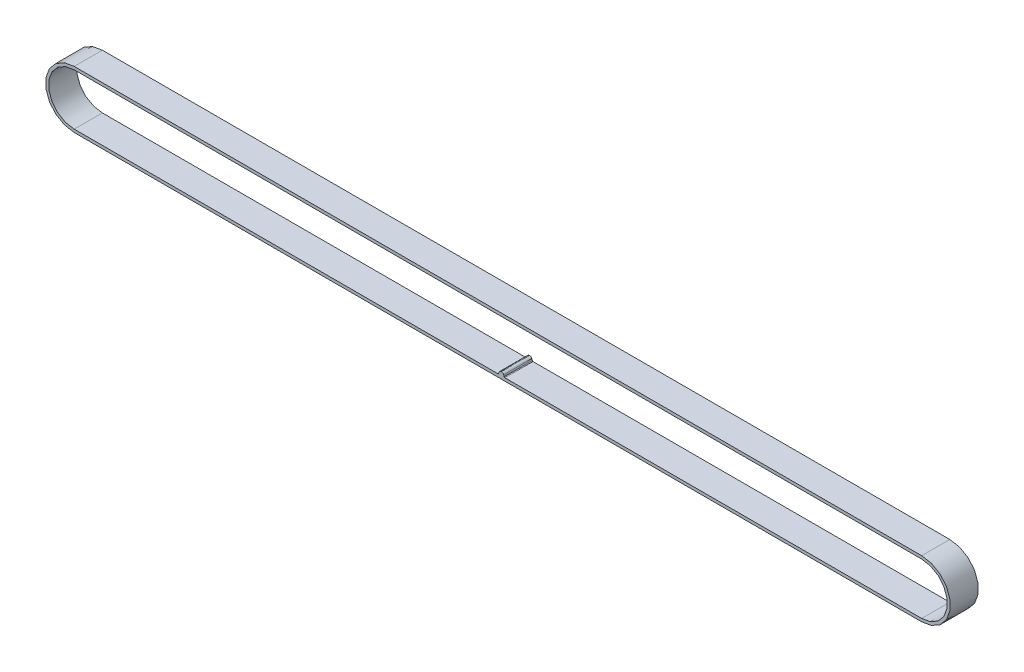
# Autodesk Inventor part: correia
Saved by Autodesk Inventor 2023 (Build 270158000, 158)
## iProperties
Created: 2022-10-19
Part Number: correia
Material: Generic
Document SubType Name: Modeling
Designer: klebe
Density: 1 g/cm^3
Appearance: Default
Author: klebe
Autodesk Inventor part; units mm, degrees
(part 1 of 6)
ref_plane "YZ Plane" through (0, 0, 0) normal (1, 0, 0) x (0, 1, 0)
ref_plane "XZ Plane" through (0, 0, 0) normal (0, 1, 0) x (-1, 0, 0)
ref_plane "XY Plane" through (0, 0, 0) normal (0, 0, 1) x (1, 0, 0)
ref_plane "Work Plane2" through (-56.6424, 85.638, -97) normal (0, 0, 1) x (-1, 0, 0)
sketch "Sketch2" plane through (-56.6424, 85.638, -97) normal (0, 0, 1) x (-1, 0, 0)
  arc A0 (0, 0) -> (0, 50.63) centre (0, 25.315) ccw
  line L0 (-421.46, 50.63) -> (0, 50.63)
  arc A1 (-421.46, 50.63) -> (-421.46, 0) centre (-421.46, 25.315) ccw
  line L1 (0, 0) -> (-421.46, 0)
  arc A2 (-204.9902, 50) -> (-205.1389, 49.8696) centre (-204.9902, 49.85) ccw
  line L2 (-204.9902, 50) -> (-204.4709, 50)
  arc A3 (-204.3222, 49.8696) -> (-204.4709, 50) centre (-204.4709, 49.85) ccw
  arc A4 (-204.3222, 49.8696) -> (-204.2296, 49.5618) centre (-203.3307, 50) ccw
  arc A5 (-204.2296, 49.5618) -> (-203.7306, 49.25) centre (-203.7307, 49.805) ccw
  arc A6 (-203.7306, 49.25) -> (-203.2315, 49.5618) centre (-203.7304, 49.805) ccw
  arc A7 (-203.2315, 49.5618) -> (-203.1389, 49.8696) centre (-204.1304, 50) ccw
  arc A8 (-202.9902, 50) -> (-203.1389, 49.8696) centre (-202.9902, 49.85) ccw
  line L3 (-202.9902, 50) -> (-202.4709, 50)
  arc A9 (-202.3222, 49.8696) -> (-202.4709, 50) centre (-202.4709, 49.85) ccw
  arc A10 (-202.3222, 49.8696) -> (-202.2296, 49.5618) centre (-201.3307, 50) ccw
  arc A11 (-202.2296, 49.5618) -> (-201.7306, 49.25) centre (-201.7307, 49.805) ccw
  arc A12 (-201.7306, 49.25) -> (-201.2315, 49.5618) centre (-201.7304, 49.805) ccw
  arc A13 (-201.2315, 49.5618) -> (-201.1389, 49.8696) centre (-202.1304, 50) ccw
  arc A14 (-200.9902, 50) -> (-201.1389, 49.8696) centre (-200.9902, 49.85) ccw
  line L4 (-200.9902, 50) -> (-200.4709, 50)
  arc A15 (-200.3222, 49.8696) -> (-200.4709, 50) centre (-200.4709, 49.85) ccw
  arc A16 (-200.3222, 49.8696) -> (-200.2296, 49.5618) centre (-199.3307, 50) ccw
  arc A17 (-200.2296, 49.5618) -> (-199.7306, 49.25) centre (-199.7307, 49.805) ccw
  arc A18 (-199.7306, 49.25) -> (-199.2315, 49.5618) centre (-199.7304, 49.805) ccw
  arc A19 (-199.2315, 49.5618) -> (-199.1389, 49.8696) centre (-200.1304, 50) ccw
  arc A20 (-198.9902, 50) -> (-199.1389, 49.8696) centre (-198.9902, 49.85) ccw
  line L5 (-198.9902, 50) -> (-198.4709, 50)
  arc A21 (-198.3222, 49.8696) -> (-198.4709, 50) centre (-198.4709, 49.85) ccw
  arc A22 (-198.3222, 49.8696) -> (-198.2296, 49.5618) centre (-197.3307, 50) ccw
  arc A23 (-198.2296, 49.5618) -> (-197.7306, 49.25) centre (-197.7307, 49.805) ccw
  arc A24 (-197.7306, 49.25) -> (-197.2315, 49.5618) centre (-197.7304, 49.805) ccw
  arc A25 (-197.2315, 49.5618) -> (-197.1389, 49.8696) centre (-198.1304, 50) ccw
  arc A26 (-196.9902, 50) -> (-197.1389, 49.8696) centre (-196.9902, 49.85) ccw
  line L6 (-196.9902, 50) -> (-196.4709, 50)
  arc A27 (-196.3222, 49.8696) -> (-196.4709, 50) centre (-196.4709, 49.85) ccw
  arc A28 (-196.3222, 49.8696) -> (-196.2296, 49.5618) centre (-195.3307, 50) ccw
  arc A29 (-196.2296, 49.5618) -> (-195.7306, 49.25) centre (-195.7307, 49.805) ccw
  arc A30 (-195.7306, 49.25) -> (-195.2315, 49.5618) centre (-195.7304, 49.805) ccw
  arc A31 (-195.2315, 49.5618) -> (-195.1389, 49.8696) centre (-196.1304, 50) ccw
  arc A32 (-194.9902, 50) -> (-195.1389, 49.8696) centre (-194.9902, 49.85) ccw
  line L7 (-194.9902, 50) -> (-194.4709, 50)
  arc A33 (-194.3222, 49.8696) -> (-194.4709, 50) centre (-194.4709, 49.85) ccw
  arc A34 (-194.3222, 49.8696) -> (-194.2296, 49.5618) centre (-193.3307, 50) ccw
  arc A35 (-194.2296, 49.5618) -> (-193.7306, 49.25) centre (-193.7307, 49.805) ccw
  arc A36 (-193.7306, 49.25) -> (-193.2315, 49.5618) centre (-193.7304, 49.805) ccw
  arc A37 (-193.2315, 49.5618) -> (-193.1389, 49.8696) centre (-194.1304, 50) ccw
  arc A38 (-192.9902, 50) -> (-193.1389, 49.8696) centre (-192.9902, 49.85) ccw
  line L8 (-192.9902, 50) -> (-192.4709, 50)
  arc A39 (-192.3222, 49.8696) -> (-192.4709, 50) centre (-192.4709, 49.85) ccw
  arc A40 (-192.3222, 49.8696) -> (-192.2296, 49.5618) centre (-191.3307, 50) ccw
  arc A41 (-192.2296, 49.5618) -> (-191.7306, 49.25) centre (-191.7307, 49.805) ccw
  arc A42 (-191.7306, 49.25) -> (-191.2315, 49.5618) centre (-191.7304, 49.805) ccw
  arc A43 (-191.2315, 49.5618) -> (-191.1389, 49.8696) centre (-192.1304, 50) ccw
  arc A44 (-190.9902, 50) -> (-191.1389, 49.8696) centre (-190.9902, 49.85) ccw
  line L9 (-190.9902, 50) -> (-190.4709, 50)
  arc A45 (-190.3222, 49.8696) -> (-190.4709, 50) centre (-190.4709, 49.85) ccw
  arc A46 (-190.3222, 49.8696) -> (-190.2296, 49.5618) centre (-189.3307, 50) ccw
  arc A47 (-190.2296, 49.5618) -> (-189.7306, 49.25) centre (-189.7307, 49.805) ccw
  arc A48 (-189.7306, 49.25) -> (-189.2315, 49.5618) centre (-189.7304, 49.805) ccw
  arc A49 (-189.2315, 49.5618) -> (-189.1389, 49.8696) centre (-190.1304, 50) ccw
  arc A50 (-188.9902, 50) -> (-189.1389, 49.8696) centre (-188.9902, 49.85) ccw
  line L10 (-188.9902, 50) -> (-188.4709, 50)
  arc A51 (-188.3222, 49.8696) -> (-188.4709, 50) centre (-188.4709, 49.85) ccw
  arc A52 (-188.3222, 49.8696) -> (-188.2296, 49.5618) centre (-187.3307, 50) ccw
  arc A53 (-188.2296, 49.5618) -> (-187.7306, 49.25) centre (-187.7307, 49.805) ccw
  arc A54 (-187.7306, 49.25) -> (-187.2315, 49.5618) centre (-187.7304, 49.805) ccw
  arc A55 (-187.2315, 49.5618) -> (-187.1389, 49.8696) centre (-188.1304, 50) ccw
  arc A56 (-186.9902, 50) -> (-187.1389, 49.8696) centre (-186.9902, 49.85) ccw
  line L11 (-186.9902, 50) -> (-186.4709, 50)
  arc A57 (-186.3222, 49.8696) -> (-186.4709, 50) centre (-186.4709, 49.85) ccw
  arc A58 (-186.3222, 49.8696) -> (-186.2296, 49.5618) centre (-185.3307, 50) ccw
  arc A59 (-186.2296, 49.5618) -> (-185.7306, 49.25) centre (-185.7307, 49.805) ccw
  arc A60 (-185.7306, 49.25) -> (-185.2315, 49.5618) centre (-185.7304, 49.805) ccw
  arc A61 (-185.2315, 49.5618) -> (-185.1389, 49.8696) centre (-186.1304, 50) ccw
  arc A62 (-184.9902, 50) -> (-185.1389, 49.8696) centre (-184.9902, 49.85) ccw
  line L12 (-184.9902, 50) -> (-184.4709, 50)
  arc A63 (-184.3222, 49.8696) -> (-184.4709, 50) centre (-184.4709, 49.85) ccw
  arc A64 (-184.3222, 49.8696) -> (-184.2296, 49.5618) centre (-183.3307, 50) ccw
  arc A65 (-184.2296, 49.5618) -> (-183.7306, 49.25) centre (-183.7307, 49.805) ccw
  arc A66 (-183.7306, 49.25) -> (-183.2315, 49.5618) centre (-183.7304, 49.805) ccw
  arc A67 (-183.2315, 49.5618) -> (-183.1389, 49.8696) centre (-184.1304, 50) ccw
  arc A68 (-182.9902, 50) -> (-183.1389, 49.8696) centre (-182.9902, 49.85) ccw
  line L13 (-182.9902, 50) -> (-182.4709, 50)
  arc A69 (-182.3222, 49.8696) -> (-182.4709, 50) centre (-182.4709, 49.85) ccw
  arc A70 (-182.3222, 49.8696) -> (-182.2296, 49.5618) centre (-181.3307, 50) ccw
  arc A71 (-182.2296, 49.5618) -> (-181.7306, 49.25) centre (-181.7307, 49.805) ccw
  arc A72 (-181.7306, 49.25) -> (-181.2315, 49.5618) centre (-181.7304, 49.805) ccw
  arc A73 (-181.2315, 49.5618) -> (-181.1389, 49.8696) centre (-182.1304, 50) ccw
  arc A74 (-180.9902, 50) -> (-181.1389, 49.8696) centre (-180.9902, 49.85) ccw
  line L14 (-180.9902, 50) -> (-180.4709, 50)
  arc A75 (-180.3222, 49.8696) -> (-180.4709, 50) centre (-180.4709, 49.85) ccw
  arc A76 (-180.3222, 49.8696) -> (-180.2296, 49.5618) centre (-179.3307, 50) ccw
  arc A77 (-180.2296, 49.5618) -> (-179.7306, 49.25) centre (-179.7307, 49.805) ccw
  arc A78 (-179.7306, 49.25) -> (-179.2315, 49.5618) centre (-179.7304, 49.805) ccw
  arc A79 (-179.2315, 49.5618) -> (-179.1389, 49.8696) centre (-180.1304, 50) ccw
  arc A80 (-178.9902, 50) -> (-179.1389, 49.8696) centre (-178.9902, 49.85) ccw
  line L15 (-178.9902, 50) -> (-178.4709, 50)
  arc A81 (-178.3222, 49.8696) -> (-178.4709, 50) centre (-178.4709, 49.85) ccw
  arc A82 (-178.3222, 49.8696) -> (-178.2296, 49.5618) centre (-177.3307, 50) ccw
  arc A83 (-178.2296, 49.5618) -> (-177.7306, 49.25) centre (-177.7307, 49.805) ccw
  arc A84 (-177.7306, 49.25) -> (-177.2315, 49.5618) centre (-177.7304, 49.805) ccw
  arc A85 (-177.2315, 49.5618) -> (-177.1389, 49.8696) centre (-178.1304, 50) ccw
  arc A86 (-176.9902, 50) -> (-177.1389, 49.8696) centre (-176.9902, 49.85) ccw
  line L16 (-176.9902, 50) -> (-176.4709, 50)
  arc A87 (-176.3222, 49.8696) -> (-176.4709, 50) centre (-176.4709, 49.85) ccw
  arc A88 (-176.3222, 49.8696) -> (-176.2296, 49.5618) centre (-175.3307, 50) ccw
  arc A89 (-176.2296, 49.5618) -> (-175.7306, 49.25) centre (-175.7307, 49.805) ccw
  arc A90 (-175.7306, 49.25) -> (-175.2315, 49.5618) centre (-175.7304, 49.805) ccw
  arc A91 (-175.2315, 49.5618) -> (-175.1389, 49.8696) centre (-176.1304, 50) ccw
  arc A92 (-174.9902, 50) -> (-175.1389, 49.8696) centre (-174.9902, 49.85) ccw
  line L17 (-174.9902, 50) -> (-174.4709, 50)
  arc A93 (-174.3222, 49.8696) -> (-174.4709, 50) centre (-174.4709, 49.85) ccw
  arc A94 (-174.3222, 49.8696) -> (-174.2296, 49.5618) centre (-173.3307, 50) ccw
  arc A95 (-174.2296, 49.5618) -> (-173.7306, 49.25) centre (-173.7307, 49.805) ccw
  arc A96 (-173.7306, 49.25) -> (-173.2315, 49.5618) centre (-173.7304, 49.805) ccw
  arc A97 (-173.2315, 49.5618) -> (-173.1389, 49.8696) centre (-174.1304, 50) ccw
  arc A98 (-172.9902, 50) -> (-173.1389, 49.8696) centre (-172.9902, 49.85) ccw
  line L18 (-172.9902, 50) -> (-172.4709, 50)
  arc A99 (-172.3222, 49.8696) -> (-172.4709, 50) centre (-172.4709, 49.85) ccw
  arc A100 (-172.3222, 49.8696) -> (-172.2296, 49.5618) centre (-171.3307, 50) ccw
  arc A101 (-172.2296, 49.5618) -> (-171.7306, 49.25) centre (-171.7307, 49.805) ccw
  arc A102 (-171.7306, 49.25) -> (-171.2315, 49.5618) centre (-171.7304, 49.805) ccw
  arc A103 (-171.2315, 49.5618) -> (-171.1389, 49.8696) centre (-172.1304, 50) ccw
  arc A104 (-170.9902, 50) -> (-171.1389, 49.8696) centre (-170.9902, 49.85) ccw
  line L19 (-170.9902, 50) -> (-170.4709, 50)
  arc A105 (-170.3222, 49.8696) -> (-170.4709, 50) centre (-170.4709, 49.85) ccw
  arc A106 (-170.3222, 49.8696) -> (-170.2296, 49.5618) centre (-169.3307, 50) ccw
  arc A107 (-170.2296, 49.5618) -> (-169.7306, 49.25) centre (-169.7307, 49.805) ccw
  arc A108 (-169.7306, 49.25) -> (-169.2315, 49.5618) centre (-169.7304, 49.805) ccw
  arc A109 (-169.2315, 49.5618) -> (-169.1389, 49.8696) centre (-170.1304, 50) ccw
  arc A110 (-168.9902, 50) -> (-169.1389, 49.8696) centre (-168.9902, 49.85) ccw
  line L20 (-168.9902, 50) -> (-168.4709, 50)
  arc A111 (-168.3222, 49.8696) -> (-168.4709, 50) centre (-168.4709, 49.85) ccw
  arc A112 (-168.3222, 49.8696) -> (-168.2296, 49.5618) centre (-167.3307, 50) ccw
  arc A113 (-168.2296, 49.5618) -> (-167.7306, 49.25) centre (-167.7307, 49.805) ccw
  arc A114 (-167.7306, 49.25) -> (-167.2315, 49.5618) centre (-167.7304, 49.805) ccw
  arc A115 (-167.2315, 49.5618) -> (-167.1389, 49.8696) centre (-168.1304, 50) ccw
  arc A116 (-166.9902, 50) -> (-167.1389, 49.8696) centre (-166.9902, 49.85) ccw
  line L21 (-166.9902, 50) -> (-166.4709, 50)
  arc A117 (-166.3222, 49.8696) -> (-166.4709, 50) centre (-166.4709, 49.85) ccw
  arc A118 (-166.3222, 49.8696) -> (-166.2296, 49.5618) centre (-165.3307, 50) ccw
  arc A119 (-166.2296, 49.5618) -> (-165.7306, 49.25) centre (-165.7307, 49.805) ccw
  arc A120 (-165.7306, 49.25) -> (-165.2315, 49.5618) centre (-165.7304, 49.805) ccw
  arc A121 (-165.2315, 49.5618) -> (-165.1389, 49.8696) centre (-166.1304, 50) ccw
  arc A122 (-164.9902, 50) -> (-165.1389, 49.8696) centre (-164.9902, 49.85) ccw
  line L22 (-164.9902, 50) -> (-164.4709, 50)
  arc A123 (-164.3222, 49.8696) -> (-164.4709, 50) centre (-164.4709, 49.85) ccw
  arc A124 (-164.3222, 49.8696) -> (-164.2296, 49.5618) centre (-163.3307, 50) ccw
  arc A125 (-164.2296, 49.5618) -> (-163.7306, 49.25) centre (-163.7307, 49.805) ccw
  arc A126 (-163.7306, 49.25) -> (-163.2315, 49.5618) centre (-163.7304, 49.805) ccw
  arc A127 (-163.2315, 49.5618) -> (-163.1389, 49.8696) centre (-164.1304, 50) ccw
  arc A128 (-162.9902, 50) -> (-163.1389, 49.8696) centre (-162.9902, 49.85) ccw
  line L23 (-162.9902, 50) -> (-162.4709, 50)
  arc A129 (-162.3222, 49.8696) -> (-162.4709, 50) centre (-162.4709, 49.85) ccw
  arc A130 (-162.3222, 49.8696) -> (-162.2296, 49.5618) centre (-161.3307, 50) ccw
  arc A131 (-162.2296, 49.5618) -> (-161.7306, 49.25) centre (-161.7307, 49.805) ccw
  arc A132 (-161.7306, 49.25) -> (-161.2315, 49.5618) centre (-161.7304, 49.805) ccw
  arc A133 (-161.2315, 49.5618) -> (-161.1389, 49.8696) centre (-162.1304, 50) ccw
  arc A134 (-160.9902, 50) -> (-161.1389, 49.8696) centre (-160.9902, 49.85) ccw
  line L24 (-160.9902, 50) -> (-160.4709, 50)
  arc A135 (-160.3222, 49.8696) -> (-160.4709, 50) centre (-160.4709, 49.85) ccw
  arc A136 (-160.3222, 49.8696) -> (-160.2296, 49.5618) centre (-159.3307, 50) ccw
  arc A137 (-160.2296, 49.5618) -> (-159.7306, 49.25) centre (-159.7307, 49.805) ccw
  arc A138 (-159.7306, 49.25) -> (-159.2315, 49.5618) centre (-159.7304, 49.805) ccw
  arc A139 (-159.2315, 49.5618) -> (-159.1389, 49.8696) centre (-160.1304, 50) ccw
  arc A140 (-158.9902, 50) -> (-159.1389, 49.8696) centre (-158.9902, 49.85) ccw
  line L25 (-158.9902, 50) -> (-158.4709, 50)
  arc A141 (-158.3222, 49.8696) -> (-158.4709, 50) centre (-158.4709, 49.85) ccw
  arc A142 (-158.3222, 49.8696) -> (-158.2296, 49.5618) centre (-157.3307, 50) ccw
  arc A143 (-158.2296, 49.5618) -> (-157.7306, 49.25) centre (-157.7307, 49.805) ccw
  arc A144 (-157.7306, 49.25) -> (-157.2315, 49.5618) centre (-157.7304, 49.805) ccw
  arc A145 (-157.2315, 49.5618) -> (-157.1389, 49.8696) centre (-158.1304, 50) ccw
  arc A146 (-156.9902, 50) -> (-157.1389, 49.8696) centre (-156.9902, 49.85) ccw
  line L26 (-156.9902, 50) -> (-156.4709, 50)
  arc A147 (-156.3222, 49.8696) -> (-156.4709, 50) centre (-156.4709, 49.85) ccw
  arc A148 (-156.3222, 49.8696) -> (-156.2296, 49.5618) centre (-155.3307, 50) ccw
  arc A149 (-156.2296, 49.5618) -> (-155.7306, 49.25) centre (-155.7307, 49.805) ccw
  arc A150 (-155.7306, 49.25) -> (-155.2315, 49.5618) centre (-155.7304, 49.805) ccw
  arc A151 (-155.2315, 49.5618) -> (-155.1389, 49.8696) centre (-156.1304, 50) ccw
  arc A152 (-154.9902, 50) -> (-155.1389, 49.8696) centre (-154.9902, 49.85) ccw
  line L27 (-154.9902, 50) -> (-154.4709, 50)
  arc A153 (-154.3222, 49.8696) -> (-154.4709, 50) centre (-154.4709, 49.85) ccw
  arc A154 (-154.3222, 49.8696) -> (-154.2296, 49.5618) centre (-153.3307, 50) ccw
  arc A155 (-154.2296, 49.5618) -> (-153.7306, 49.25) centre (-153.7307, 49.805) ccw
  arc A156 (-153.7306, 49.25) -> (-153.2315, 49.5618) centre (-153.7304, 49.805) ccw
  arc A157 (-153.2315, 49.5618) -> (-153.1389, 49.8696) centre (-154.1304, 50) ccw
  arc A158 (-152.9902, 50) -> (-153.1389, 49.8696) centre (-152.9902, 49.85) ccw
  line L28 (-152.9902, 50) -> (-152.4709, 50)
  arc A159 (-152.3222, 49.8696) -> (-152.4709, 50) centre (-152.4709, 49.85) ccw
  arc A160 (-152.3222, 49.8696) -> (-152.2296, 49.5618) centre (-151.3307, 50) ccw
  arc A161 (-152.2296, 49.5618) -> (-151.7306, 49.25) centre (-151.7307, 49.805) ccw
  arc A162 (-151.7306, 49.25) -> (-151.2315, 49.5618) centre (-151.7304, 49.805) ccw
  arc A163 (-151.2315, 49.5618) -> (-151.1389, 49.8696) centre (-152.1304, 50) ccw
  arc A164 (-150.9902, 50) -> (-151.1389, 49.8696) centre (-150.9902, 49.85) ccw
  line L29 (-150.9902, 50) -> (-150.4709, 50)
  arc A165 (-150.3222, 49.8696) -> (-150.4709, 50) centre (-150.4709, 49.85) ccw
  arc A166 (-150.3222, 49.8696) -> (-150.2296, 49.5618) centre (-149.3307, 50) ccw
  arc A167 (-150.2296, 49.5618) -> (-149.7306, 49.25) centre (-149.7307, 49.805) ccw
  arc A168 (-149.7306, 49.25) -> (-149.2315, 49.5618) centre (-149.7304, 49.805) ccw
  arc A169 (-149.2315, 49.5618) -> (-149.1389, 49.8696) centre (-150.1304, 50) ccw
  arc A170 (-148.9902, 50) -> (-149.1389, 49.8696) centre (-148.9902, 49.85) ccw
  line L30 (-148.9902, 50) -> (-148.4709, 50)
  arc A171 (-148.3222, 49.8696) -> (-148.4709, 50) centre (-148.4709, 49.85) ccw
  arc A172 (-148.3222, 49.8696) -> (-148.2296, 49.5618) centre (-147.3307, 50) ccw
  arc A173 (-148.2296, 49.5618) -> (-147.7306, 49.25) centre (-147.7307, 49.805) ccw
  arc A174 (-147.7306, 49.25) -> (-147.2315, 49.5618) centre (-147.7304, 49.805) ccw
  arc A175 (-147.2315, 49.5618) -> (-147.1389, 49.8696) centre (-148.1304, 50) ccw
  arc A176 (-146.9902, 50) -> (-147.1389, 49.8696) centre (-146.9902, 49.85) ccw
  line L31 (-146.9902, 50) -> (-146.4709, 50)
  arc A177 (-146.3222, 49.8696) -> (-146.4709, 50) centre (-146.4709, 49.85) ccw
  arc A178 (-146.3222, 49.8696) -> (-146.2296, 49.5618) centre (-145.3307, 50) ccw
  arc A179 (-146.2296, 49.5618) -> (-145.7306, 49.25) centre (-145.7307, 49.805) ccw
  arc A180 (-145.7306, 49.25) -> (-145.2315, 49.5618) centre (-145.7304, 49.805) ccw
  arc A181 (-145.2315, 49.5618) -> (-145.1389, 49.8696) centre (-146.1304, 50) ccw
  arc A182 (-144.9902, 50) -> (-145.1389, 49.8696) centre (-144.9902, 49.85) ccw
  line L32 (-144.9902, 50) -> (-144.4709, 50)
  arc A183 (-144.3222, 49.8696) -> (-144.4709, 50) centre (-144.4709, 49.85) ccw
  arc A184 (-144.3222, 49.8696) -> (-144.2296, 49.5618) centre (-143.3307, 50) ccw
  arc A185 (-144.2296, 49.5618) -> (-143.7306, 49.25) centre (-143.7307, 49.805) ccw
  arc A186 (-143.7306, 49.25) -> (-143.2315, 49.5618) centre (-143.7304, 49.805) ccw
  arc A187 (-143.2315, 49.5618) -> (-143.1389, 49.8696) centre (-144.1304, 50) ccw
  arc A188 (-142.9902, 50) -> (-143.1389, 49.8696) centre (-142.9902, 49.85) ccw
  line L33 (-142.9902, 50) -> (-142.4709, 50)
  arc A189 (-142.3222, 49.8696) -> (-142.4709, 50) centre (-142.4709, 49.85) ccw
  arc A190 (-142.3222, 49.8696) -> (-142.2296, 49.5618) centre (-141.3307, 50) ccw
  arc A191 (-142.2296, 49.5618) -> (-141.7306, 49.25) centre (-141.7307, 49.805) ccw
  arc A192 (-141.7306, 49.25) -> (-141.2315, 49.5618) centre (-141.7304, 49.805) ccw
  arc A193 (-141.2315, 49.5618) -> (-141.1389, 49.8696) centre (-142.1304, 50) ccw
  arc A194 (-140.9902, 50) -> (-141.1389, 49.8696) centre (-140.9902, 49.85) ccw
  line L34 (-140.9902, 50) -> (-140.4709, 50)
  arc A195 (-140.3222, 49.8696) -> (-140.4709, 50) centre (-140.4709, 49.85) ccw
  arc A196 (-140.3222, 49.8696) -> (-140.2296, 49.5618) centre (-139.3307, 50) ccw
  arc A197 (-140.2296, 49.5618) -> (-139.7306, 49.25) centre (-139.7307, 49.805) ccw
  arc A198 (-139.7306, 49.25) -> (-139.2315, 49.5618) centre (-139.7304, 49.805) ccw
  arc A199 (-139.2315, 49.5618) -> (-139.1389, 49.8696) centre (-140.1304, 50) ccw
  arc A200 (-138.9902, 50) -> (-139.1389, 49.8696) centre (-138.9902, 49.85) ccw
  line L35 (-138.9902, 50) -> (-138.4709, 50)
  arc A201 (-138.3222, 49.8696) -> (-138.4709, 50) centre (-138.4709, 49.85) ccw
  arc A202 (-138.3222, 49.8696) -> (-138.2296, 49.5618) centre (-137.3307, 50) ccw
  arc A203 (-138.2296, 49.5618) -> (-137.7306, 49.25) centre (-137.7307, 49.805) ccw
  arc A204 (-137.7306, 49.25) -> (-137.2315, 49.5618) centre (-137.7304, 49.805) ccw
  arc A205 (-137.2315, 49.5618) -> (-137.1389, 49.8696) centre (-138.1304, 50) ccw
  arc A206 (-136.9902, 50) -> (-137.1389, 49.8696) centre (-136.9902, 49.85) ccw
  line L36 (-136.9902, 50) -> (-136.4709, 50)
  arc A207 (-136.3222, 49.8696) -> (-136.4709, 50) centre (-136.4709, 49.85) ccw
  arc A208 (-136.3222, 49.8696) -> (-136.2296, 49.5618) centre (-135.3307, 50) ccw
  arc A209 (-136.2296, 49.5618) -> (-135.7306, 49.25) centre (-135.7307, 49.805) ccw
  arc A210 (-135.7306, 49.25) -> (-135.2315, 49.5618) centre (-135.7304, 49.805) ccw
  arc A211 (-135.2315, 49.5618) -> (-135.1389, 49.8696) centre (-136.1304, 50) ccw
  arc A212 (-134.9902, 50) -> (-135.1389, 49.8696) centre (-134.9902, 49.85) ccw
  line L37 (-134.9902, 50) -> (-134.4709, 50)
  arc A213 (-134.3222, 49.8696) -> (-134.4709, 50) centre (-134.4709, 49.85) ccw
  arc A214 (-134.3222, 49.8696) -> (-134.2296, 49.5618) centre (-133.3307, 50) ccw
  arc A215 (-134.2296, 49.5618) -> (-133.7306, 49.25) centre (-133.7307, 49.805) ccw
  arc A216 (-133.7306, 49.25) -> (-133.2315, 49.5618) centre (-133.7304, 49.805) ccw
  arc A217 (-133.2315, 49.5618) -> (-133.1389, 49.8696) centre (-134.1304, 50) ccw
  arc A218 (-132.9902, 50) -> (-133.1389, 49.8696) centre (-132.9902, 49.85) ccw
  line L38 (-132.9902, 50) -> (-132.4709, 50)
  arc A219 (-132.3222, 49.8696) -> (-132.4709, 50) centre (-132.4709, 49.85) ccw
  arc A220 (-132.3222, 49.8696) -> (-132.2296, 49.5618) centre (-131.3307, 50) ccw
  arc A221 (-132.2296, 49.5618) -> (-131.7306, 49.25) centre (-131.7307, 49.805) ccw
  arc A222 (-131.7306, 49.25) -> (-131.2315, 49.5618) centre (-131.7304, 49.805) ccw
  arc A223 (-131.2315, 49.5618) -> (-131.1389, 49.8696) centre (-132.1304, 50) ccw
  arc A224 (-130.9902, 50) -> (-131.1389, 49.8696) centre (-130.9902, 49.85) ccw
  line L39 (-130.9902, 50) -> (-130.4709, 50)
  arc A225 (-130.3222, 49.8696) -> (-130.4709, 50) centre (-130.4709, 49.85) ccw
  arc A226 (-130.3222, 49.8696) -> (-130.2296, 49.5618) centre (-129.3307, 50) ccw
  arc A227 (-130.2296, 49.5618) -> (-129.7306, 49.25) centre (-129.7307, 49.805) ccw
  arc A228 (-129.7306, 49.25) -> (-129.2315, 49.5618) centre (-129.7304, 49.805) ccw
  arc A229 (-129.2315, 49.5618) -> (-129.1389, 49.8696) centre (-130.1304, 50) ccw
  arc A230 (-128.9902, 50) -> (-129.1389, 49.8696) centre (-128.9902, 49.85) ccw
  line L40 (-128.9902, 50) -> (-128.4709, 50)
  arc A231 (-128.3222, 49.8696) -> (-128.4709, 50) centre (-128.4709, 49.85) ccw
  arc A232 (-128.3222, 49.8696) -> (-128.2296, 49.5618) centre (-127.3307, 50) ccw
  arc A233 (-128.2296, 49.5618) -> (-127.7306, 49.25) centre (-127.7307, 49.805) ccw
  arc A234 (-127.7306, 49.25) -> (-127.2315, 49.5618) centre (-127.7304, 49.805) ccw
  arc A235 (-127.2315, 49.5618) -> (-127.1389, 49.8696) centre (-128.1304, 50) ccw
  arc A236 (-126.9902, 50) -> (-127.1389, 49.8696) centre (-126.9902, 49.85) ccw
  line L41 (-126.9902, 50) -> (-126.4709, 50)
  arc A237 (-126.3222, 49.8696) -> (-126.4709, 50) centre (-126.4709, 49.85) ccw
  arc A238 (-126.3222, 49.8696) -> (-126.2296, 49.5618) centre (-125.3307, 50) ccw
  arc A239 (-126.2296, 49.5618) -> (-125.7306, 49.25) centre (-125.7307, 49.805) ccw
  arc A240 (-125.7306, 49.25) -> (-125.2315, 49.5618) centre (-125.7304, 49.805) ccw
  arc A241 (-125.2315, 49.5618) -> (-125.1389, 49.8696) centre (-126.1304, 50) ccw
  arc A242 (-124.9902, 50) -> (-125.1389, 49.8696) centre (-124.9902, 49.85) ccw
  line L42 (-124.9902, 50) -> (-124.4709, 50)
  arc A243 (-124.3222, 49.8696) -> (-124.4709, 50) centre (-124.4709, 49.85) ccw
  arc A244 (-124.3222, 49.8696) -> (-124.2296, 49.5618) centre (-123.3307, 50) ccw
  arc A245 (-124.2296, 49.5618) -> (-123.7306, 49.25) centre (-123.7307, 49.805) ccw
  arc A246 (-123.7306, 49.25) -> (-123.2315, 49.5618) centre (-123.7304, 49.805) ccw
  arc A247 (-123.2315, 49.5618) -> (-123.1389, 49.8696) centre (-124.1304, 50) ccw
  arc A248 (-122.9902, 50) -> (-123.1389, 49.8696) centre (-122.9902, 49.85) ccw
  line L43 (-122.9902, 50) -> (-122.4709, 50)
  arc A249 (-122.3222, 49.8696) -> (-122.4709, 50) centre (-122.4709, 49.85) ccw
  arc A250 (-122.3222, 49.8696) -> (-122.2296, 49.5618) centre (-121.3307, 50) ccw
  arc A251 (-122.2296, 49.5618) -> (-121.7306, 49.25) centre (-121.7307, 49.805) ccw
  arc A252 (-121.7306, 49.25) -> (-121.2315, 49.5618) centre (-121.7304, 49.805) ccw
  arc A253 (-121.2315, 49.5618) -> (-121.1389, 49.8696) centre (-122.1304, 50) ccw
  arc A254 (-120.9902, 50) -> (-121.1389, 49.8696) centre (-120.9902, 49.85) ccw
  line L44 (-120.9902, 50) -> (-120.4709, 50)
  arc A255 (-120.3222, 49.8696) -> (-120.4709, 50) centre (-120.4709, 49.85) ccw
  arc A256 (-120.3222, 49.8696) -> (-120.2296, 49.5618) centre (-119.3307, 50) ccw
  arc A257 (-120.2296, 49.5618) -> (-119.7306, 49.25) centre (-119.7307, 49.805) ccw
  arc A258 (-119.7306, 49.25) -> (-119.2315, 49.5618) centre (-119.7304, 49.805) ccw
  arc A259 (-119.2315, 49.5618) -> (-119.1389, 49.8696) centre (-120.1304, 50) ccw
  arc A260 (-118.9902, 50) -> (-119.1389, 49.8696) centre (-118.9902, 49.85) ccw
  line L45 (-118.9902, 50) -> (-118.4709, 50)
  arc A261 (-118.3222, 49.8696) -> (-118.4709, 50) centre (-118.4709, 49.85) ccw
  arc A262 (-118.3222, 49.8696) -> (-118.2296, 49.5618) centre (-117.3307, 50) ccw
  arc A263 (-118.2296, 49.5618) -> (-117.7306, 49.25) centre (-117.7307, 49.805) ccw
  arc A264 (-117.7306, 49.25) -> (-117.2315, 49.5618) centre (-117.7304, 49.805) ccw
  arc A265 (-117.2315, 49.5618) -> (-117.1389, 49.8696) centre (-118.1304, 50) ccw
  arc A266 (-116.9902, 50) -> (-117.1389, 49.8696) centre (-116.9902, 49.85) ccw
  line L46 (-116.9902, 50) -> (-116.4709, 50)
  arc A267 (-116.3222, 49.8696) -> (-116.4709, 50) centre (-116.4709, 49.85) ccw
  arc A268 (-116.3222, 49.8696) -> (-116.2296, 49.5618) centre (-115.3307, 50) ccw
  arc A269 (-116.2296, 49.5618) -> (-115.7306, 49.25) centre (-115.7307, 49.805) ccw
  arc A270 (-115.7306, 49.25) -> (-115.2315, 49.5618) centre (-115.7304, 49.805) ccw
  arc A271 (-115.2315, 49.5618) -> (-115.1389, 49.8696) centre (-116.1304, 50) ccw
  arc A272 (-114.9902, 50) -> (-115.1389, 49.8696) centre (-114.9902, 49.85) ccw
  line L47 (-114.9902, 50) -> (-114.4709, 50)
  arc A273 (-114.3222, 49.8696) -> (-114.4709, 50) centre (-114.4709, 49.85) ccw
  arc A274 (-114.3222, 49.8696) -> (-114.2296, 49.5618) centre (-113.3307, 50) ccw
  arc A275 (-114.2296, 49.5618) -> (-113.7306, 49.25) centre (-113.7307, 49.805) ccw
  arc A276 (-113.7306, 49.25) -> (-113.2315, 49.5618) centre (-113.7304, 49.805) ccw
  arc A277 (-113.2315, 49.5618) -> (-113.1389, 49.8696) centre (-114.1304, 50) ccw
  arc A278 (-112.9902, 50) -> (-113.1389, 49.8696) centre (-112.9902, 49.85) ccw
  line L48 (-112.9902, 50) -> (-112.4709, 50)
  arc A279 (-112.3222, 49.8696) -> (-112.4709, 50) centre (-112.4709, 49.85) ccw
  arc A280 (-112.3222, 49.8696) -> (-112.2296, 49.5618) centre (-111.3307, 50) ccw
  arc A281 (-112.2296, 49.5618) -> (-111.7306, 49.25) centre (-111.7307, 49.805) ccw
  arc A282 (-111.7306, 49.25) -> (-111.2315, 49.5618) centre (-111.7304, 49.805) ccw
  arc A283 (-111.2315, 49.5618) -> (-111.1389, 49.8696) centre (-112.1304, 50) ccw
  arc A284 (-110.9902, 50) -> (-111.1389, 49.8696) centre (-110.9902, 49.85) ccw
  line L49 (-110.9902, 50) -> (-110.4709, 50)
  arc A285 (-110.3222, 49.8696) -> (-110.4709, 50) centre (-110.4709, 49.85) ccw
  arc A286 (-110.3222, 49.8696) -> (-110.2296, 49.5618) centre (-109.3307, 50) ccw
  arc A287 (-110.2296, 49.5618) -> (-109.7306, 49.25) centre (-109.7307, 49.805) ccw
  arc A288 (-109.7306, 49.25) -> (-109.2315, 49.5618) centre (-109.7304, 49.805) ccw
  arc A289 (-109.2315, 49.5618) -> (-109.1389, 49.8696) centre (-110.1304, 50) ccw
  arc A290 (-108.9902, 50) -> (-109.1389, 49.8696) centre (-108.9902, 49.85) ccw
  line L50 (-108.9902, 50) -> (-108.4709, 50)
  arc A291 (-108.3222, 49.8696) -> (-108.4709, 50) centre (-108.4709, 49.85) ccw
  arc A292 (-108.3222, 49.8696) -> (-108.2296, 49.5618) centre (-107.3307, 50) ccw
  arc A293 (-108.2296, 49.5618) -> (-107.7306, 49.25) centre (-107.7307, 49.805) ccw
  arc A294 (-107.7306, 49.25) -> (-107.2315, 49.5618) centre (-107.7304, 49.805) ccw
  arc A295 (-107.2315, 49.5618) -> (-107.1389, 49.8696) centre (-108.1304, 50) ccw
  arc A296 (-106.9902, 50) -> (-107.1389, 49.8696) centre (-106.9902, 49.85) ccw
  line L51 (-106.9902, 50) -> (-106.4709, 50)
  arc A297 (-106.3222, 49.8696) -> (-106.4709, 50) centre (-106.4709, 49.85) ccw
  arc A298 (-106.3222, 49.8696) -> (-106.2296, 49.5618) centre (-105.3307, 50) ccw
  arc A299 (-106.2296, 49.5618) -> (-105.7306, 49.25) centre (-105.7307, 49.805) ccw
  arc A300 (-105.7306, 49.25) -> (-105.2315, 49.5618) centre (-105.7304, 49.805) ccw
  arc A301 (-105.2315, 49.5618) -> (-105.1389, 49.8696) centre (-106.1304, 50) ccw
  arc A302 (-104.9902, 50) -> (-105.1389, 49.8696) centre (-104.9902, 49.85) ccw
  line L52 (-104.9902, 50) -> (-104.4709, 50)
  arc A303 (-104.3222, 49.8696) -> (-104.4709, 50) centre (-104.4709, 49.85) ccw
  arc A304 (-104.3222, 49.8696) -> (-104.2296, 49.5618) centre (-103.3307, 50) ccw
  arc A305 (-104.2296, 49.5618) -> (-103.7306, 49.25) centre (-103.7307, 49.805) ccw
  arc A306 (-103.7306, 49.25) -> (-103.2315, 49.5618) centre (-103.7304, 49.805) ccw
  arc A307 (-103.2315, 49.5618) -> (-103.1389, 49.8696) centre (-104.1304, 50) ccw
  arc A308 (-102.9902, 50) -> (-103.1389, 49.8696) centre (-102.9902, 49.85) ccw
  line L53 (-102.9902, 50) -> (-102.4709, 50)
  arc A309 (-102.3222, 49.8696) -> (-102.4709, 50) centre (-102.4709, 49.85) ccw
  arc A310 (-102.3222, 49.8696) -> (-102.2296, 49.5618) centre (-101.3307, 50) ccw
  arc A311 (-102.2296, 49.5618) -> (-101.7306, 49.25) centre (-101.7307, 49.805) ccw
  arc A312 (-101.7306, 49.25) -> (-101.2315, 49.5618) centre (-101.7304, 49.805) ccw
  arc A313 (-101.2315, 49.5618) -> (-101.1389, 49.8696) centre (-102.1304, 50) ccw
  arc A314 (-100.9902, 50) -> (-101.1389, 49.8696) centre (-100.9902, 49.85) ccw
  line L54 (-100.9902, 50) -> (-100.4709, 50)
  arc A315 (-100.3222, 49.8696) -> (-100.4709, 50) centre (-100.4709, 49.85) ccw
  arc A316 (-100.3222, 49.8696) -> (-100.2296, 49.5618) centre (-99.3307, 50) ccw
  arc A317 (-100.2296, 49.5618) -> (-99.7306, 49.25) centre (-99.7307, 49.805) ccw
  arc A318 (-99.7306, 49.25) -> (-99.2315, 49.5618) centre (-99.7304, 49.805) ccw
  arc A319 (-99.2315, 49.5618) -> (-99.1389, 49.8696) centre (-100.1304, 50) ccw
  arc A320 (-98.9902, 50) -> (-99.1389, 49.8696) centre (-98.9902, 49.85) ccw
  line L55 (-98.9902, 50) -> (-98.4709, 50)
  arc A321 (-98.3222, 49.8696) -> (-98.4709, 50) centre (-98.4709, 49.85) ccw
  arc A322 (-98.3222, 49.8696) -> (-98.2296, 49.5618) centre (-97.3307, 50) ccw
  arc A323 (-98.2296, 49.5618) -> (-97.7306, 49.25) centre (-97.7307, 49.805) ccw
  arc A324 (-97.7306, 49.25) -> (-97.2315, 49.5618) centre (-97.7304, 49.805) ccw
  arc A325 (-97.2315, 49.5618) -> (-97.1389, 49.8696) centre (-98.1304, 50) ccw
  arc A326 (-96.9902, 50) -> (-97.1389, 49.8696) centre (-96.9902, 49.85) ccw
  line L56 (-96.9902, 50) -> (-96.4709, 50)
  arc A327 (-96.3222, 49.8696) -> (-96.4709, 50) centre (-96.4709, 49.85) ccw
  arc A328 (-96.3222, 49.8696) -> (-96.2296, 49.5618) centre (-95.3307, 50) ccw
  arc A329 (-96.2296, 49.5618) -> (-95.7306, 49.25) centre (-95.7307, 49.805) ccw
  arc A330 (-95.7306, 49.25) -> (-95.2315, 49.5618) centre (-95.7304, 49.805) ccw
  arc A331 (-95.2315, 49.5618) -> (-95.1389, 49.8696) centre (-96.1304, 50) ccw
  arc A332 (-94.9902, 50) -> (-95.1389, 49.8696) centre (-94.9902, 49.85) ccw
  line L57 (-94.9902, 50) -> (-94.4709, 50)
  arc A333 (-94.3222, 49.8696) -> (-94.4709, 50) centre (-94.4709, 49.85) ccw
  arc A334 (-94.3222, 49.8696) -> (-94.2296, 49.5618) centre (-93.3307, 50) ccw
  arc A335 (-94.2296, 49.5618) -> (-93.7306, 49.25) centre (-93.7307, 49.805) ccw
  arc A336 (-93.7306, 49.25) -> (-93.2315, 49.5618) centre (-93.7304, 49.805) ccw
  arc A337 (-93.2315, 49.5618) -> (-93.1389, 49.8696) centre (-94.1304, 50) ccw
  arc A338 (-92.9902, 50) -> (-93.1389, 49.8696) centre (-92.9902, 49.85) ccw
  line L58 (-92.9902, 50) -> (-92.4709, 50)
  arc A339 (-92.3222, 49.8696) -> (-92.4709, 50) centre (-92.4709, 49.85) ccw
  arc A340 (-92.3222, 49.8696) -> (-92.2296, 49.5618) centre (-91.3307, 50) ccw
  arc A341 (-92.2296, 49.5618) -> (-91.7306, 49.25) centre (-91.7307, 49.805) ccw
  arc A342 (-91.7306, 49.25) -> (-91.2315, 49.5618) centre (-91.7304, 49.805) ccw
  arc A343 (-91.2315, 49.5618) -> (-91.1389, 49.8696) centre (-92.1304, 50) ccw
  arc A344 (-90.9902, 50) -> (-91.1389, 49.8696) centre (-90.9902, 49.85) ccw
  line L59 (-90.9902, 50) -> (-90.4709, 50)
  arc A345 (-90.3222, 49.8696) -> (-90.4709, 50) centre (-90.4709, 49.85) ccw
  arc A346 (-90.3222, 49.8696) -> (-90.2296, 49.5618) centre (-89.3307, 50) ccw
  arc A347 (-90.2296, 49.5618) -> (-89.7306, 49.25) centre (-89.7307, 49.805) ccw
  arc A348 (-89.7306, 49.25) -> (-89.2315, 49.5618) centre (-89.7304, 49.805) ccw
  arc A349 (-89.2315, 49.5618) -> (-89.1389, 49.8696) centre (-90.1304, 50) ccw
  arc A350 (-88.9902, 50) -> (-89.1389, 49.8696) centre (-88.9902, 49.85) ccw
  line L60 (-88.9902, 50) -> (-88.4709, 50)
  arc A351 (-88.3222, 49.8696) -> (-88.4709, 50) centre (-88.4709, 49.85) ccw
  arc A352 (-88.3222, 49.8696) -> (-88.2296, 49.5618) centre (-87.3307, 50) ccw
  arc A353 (-88.2296, 49.5618) -> (-87.7306, 49.25) centre (-87.7307, 49.805) ccw
  arc A354 (-87.7306, 49.25) -> (-87.2315, 49.5618) centre (-87.7304, 49.805) ccw
  arc A355 (-87.2315, 49.5618) -> (-87.1389, 49.8696) centre (-88.1304, 50) ccw
  arc A356 (-86.9902, 50) -> (-87.1389, 49.8696) centre (-86.9902, 49.85) ccw
  line L61 (-86.9902, 50) -> (-86.4709, 50)
  arc A357 (-86.3222, 49.8696) -> (-86.4709, 50) centre (-86.4709, 49.85) ccw
  arc A358 (-86.3222, 49.8696) -> (-86.2296, 49.5618) centre (-85.3307, 50) ccw
  arc A359 (-86.2296, 49.5618) -> (-85.7306, 49.25) centre (-85.7307, 49.805) ccw
  arc A360 (-85.7306, 49.25) -> (-85.2315, 49.5618) centre (-85.7304, 49.805) ccw
  arc A361 (-85.2315, 49.5618) -> (-85.1389, 49.8696) centre (-86.1304, 50) ccw
  arc A362 (-84.9902, 50) -> (-85.1389, 49.8696) centre (-84.9902, 49.85) ccw
  line L62 (-84.9902, 50) -> (-84.4709, 50)
  arc A363 (-84.3222, 49.8696) -> (-84.4709, 50) centre (-84.4709, 49.85) ccw
  arc A364 (-84.3222, 49.8696) -> (-84.2296, 49.5618) centre (-83.3307, 50) ccw
  arc A365 (-84.2296, 49.5618) -> (-83.7306, 49.25) centre (-83.7307, 49.805) ccw
  arc A366 (-83.7306, 49.25) -> (-83.2315, 49.5618) centre (-83.7304, 49.805) ccw
  arc A367 (-83.2315, 49.5618) -> (-83.1389, 49.8696) centre (-84.1304, 50) ccw
  arc A368 (-82.9902, 50) -> (-83.1389, 49.8696) centre (-82.9902, 49.85) ccw
  line L63 (-82.9902, 50) -> (-82.4709, 50)
  arc A369 (-82.3222, 49.8696) -> (-82.4709, 50) centre (-82.4709, 49.85) ccw
  arc A370 (-82.3222, 49.8696) -> (-82.2296, 49.5618) centre (-81.3307, 50) ccw
  arc A371 (-82.2296, 49.5618) -> (-81.7306, 49.25) centre (-81.7307, 49.805) ccw
  arc A372 (-81.7306, 49.25) -> (-81.2315, 49.5618) centre (-81.7304, 49.805) ccw
  arc A373 (-81.2315, 49.5618) -> (-81.1389, 49.8696) centre (-82.1304, 50) ccw
  arc A374 (-80.9902, 50) -> (-81.1389, 49.8696) centre (-80.9902, 49.85) ccw
  line L64 (-80.9902, 50) -> (-80.4709, 50)
  arc A375 (-80.3222, 49.8696) -> (-80.4709, 50) centre (-80.4709, 49.85) ccw
  arc A376 (-80.3222, 49.8696) -> (-80.2296, 49.5618) centre (-79.3307, 50) ccw
  arc A377 (-80.2296, 49.5618) -> (-79.7306, 49.25) centre (-79.7307, 49.805) ccw
  arc A378 (-79.7306, 49.25) -> (-79.2315, 49.5618) centre (-79.7304, 49.805) ccw
  arc A379 (-79.2315, 49.5618) -> (-79.1389, 49.8696) centre (-80.1304, 50) ccw
  arc A380 (-78.9902, 50) -> (-79.1389, 49.8696) centre (-78.9902, 49.85) ccw
  line L65 (-78.9902, 50) -> (-78.4709, 50)
  arc A381 (-78.3222, 49.8696) -> (-78.4709, 50) centre (-78.4709, 49.85) ccw
  arc A382 (-78.3222, 49.8696) -> (-78.2296, 49.5618) centre (-77.3307, 50) ccw
  arc A383 (-78.2296, 49.5618) -> (-77.7306, 49.25) centre (-77.7307, 49.805) ccw
  arc A384 (-77.7306, 49.25) -> (-77.2315, 49.5618) centre (-77.7304, 49.805) ccw
  arc A385 (-77.2315, 49.5618) -> (-77.1389, 49.8696) centre (-78.1304, 50) ccw
  arc A386 (-76.9902, 50) -> (-77.1389, 49.8696) centre (-76.9902, 49.85) ccw
  line L66 (-76.9902, 50) -> (-76.4709, 50)
  arc A387 (-76.3222, 49.8696) -> (-76.4709, 50) centre (-76.4709, 49.85) ccw
  arc A388 (-76.3222, 49.8696) -> (-76.2296, 49.5618) centre (-75.3307, 50) ccw
  arc A389 (-76.2296, 49.5618) -> (-75.7306, 49.25) centre (-75.7307, 49.805) ccw
  arc A390 (-75.7306, 49.25) -> (-75.2315, 49.5618) centre (-75.7304, 49.805) ccw
  arc A391 (-75.2315, 49.5618) -> (-75.1389, 49.8696) centre (-76.1304, 50) ccw
  arc A392 (-74.9902, 50) -> (-75.1389, 49.8696) centre (-74.9902, 49.85) ccw
  line L67 (-74.9902, 50) -> (-74.4709, 50)
  arc A393 (-74.3222, 49.8696) -> (-74.4709, 50) centre (-74.4709, 49.85) ccw
  arc A394 (-74.3222, 49.8696) -> (-74.2296, 49.5618) centre (-73.3307, 50) ccw
  arc A395 (-74.2296, 49.5618) -> (-73.7306, 49.25) centre (-73.7307, 49.805) ccw
  arc A396 (-73.7306, 49.25) -> (-73.2315, 49.5618) centre (-73.7304, 49.805) ccw
  arc A397 (-73.2315, 49.5618) -> (-73.1389, 49.8696) centre (-74.1304, 50) ccw
  arc A398 (-72.9902, 50) -> (-73.1389, 49.8696) centre (-72.9902, 49.85) ccw
  line L68 (-72.9902, 50) -> (-72.4709, 50)
  arc A399 (-72.3222, 49.8696) -> (-72.4709, 50) centre (-72.4709, 49.85) ccw
  arc A400 (-72.3222, 49.8696) -> (-72.2296, 49.5618) centre (-71.3307, 50) ccw
  arc A401 (-72.2296, 49.5618) -> (-71.7306, 49.25) centre (-71.7307, 49.805) ccw
  arc A402 (-71.7306, 49.25) -> (-71.2315, 49.5618) centre (-71.7304, 49.805) ccw
  arc A403 (-71.2315, 49.5618) -> (-71.1389, 49.8696) centre (-72.1304, 50) ccw
  arc A404 (-70.9902, 50) -> (-71.1389, 49.8696) centre (-70.9902, 49.85) ccw
  line L69 (-70.9902, 50) -> (-70.4709, 50)
  arc A405 (-70.3222, 49.8696) -> (-70.4709, 50) centre (-70.4709, 49.85) ccw
  arc A406 (-70.3222, 49.8696) -> (-70.2296, 49.5618) centre (-69.3307, 50) ccw
  arc A407 (-70.2296, 49.5618) -> (-69.7306, 49.25) centre (-69.7307, 49.805) ccw
  arc A408 (-69.7306, 49.25) -> (-69.2315, 49.5618) centre (-69.7304, 49.805) ccw
  arc A409 (-69.2315, 49.5618) -> (-69.1389, 49.8696) centre (-70.1304, 50) ccw
  arc A410 (-68.9902, 50) -> (-69.1389, 49.8696) centre (-68.9902, 49.85) ccw
  line L70 (-68.9902, 50) -> (-68.4709, 50)
  arc A411 (-68.3222, 49.8696) -> (-68.4709, 50) centre (-68.4709, 49.85) ccw
  arc A412 (-68.3222, 49.8696) -> (-68.2296, 49.5618) centre (-67.3307, 50) ccw
  arc A413 (-68.2296, 49.5618) -> (-67.7306, 49.25) centre (-67.7307, 49.805) ccw
  arc A414 (-67.7306, 49.25) -> (-67.2315, 49.5618) centre (-67.7304, 49.805) ccw
  arc A415 (-67.2315, 49.5618) -> (-67.1389, 49.8696) centre (-68.1304, 50) ccw
  arc A416 (-66.9902, 50) -> (-67.1389, 49.8696) centre (-66.9902, 49.85) ccw
  line L71 (-66.9902, 50) -> (-66.4709, 50)
  arc A417 (-66.3222, 49.8696) -> (-66.4709, 50) centre (-66.4709, 49.85) ccw
  arc A418 (-66.3222, 49.8696) -> (-66.2296, 49.5618) centre (-65.3307, 50) ccw
  arc A419 (-66.2296, 49.5618) -> (-65.7306, 49.25) centre (-65.7307, 49.805) ccw
  arc A420 (-65.7306, 49.25) -> (-65.2315, 49.5618) centre (-65.7304, 49.805) ccw
  arc A421 (-65.2315, 49.5618) -> (-65.1389, 49.8696) centre (-66.1304, 50) ccw
  arc A422 (-64.9902, 50) -> (-65.1389, 49.8696) centre (-64.9902, 49.85) ccw
  line L72 (-64.9902, 50) -> (-64.4709, 50)
  arc A423 (-64.3222, 49.8696) -> (-64.4709, 50) centre (-64.4709, 49.85) ccw
  arc A424 (-64.3222, 49.8696) -> (-64.2296, 49.5618) centre (-63.3307, 50) ccw
  arc A425 (-64.2296, 49.5618) -> (-63.7306, 49.25) centre (-63.7307, 49.805) ccw
  arc A426 (-63.7306, 49.25) -> (-63.2315, 49.5618) centre (-63.7304, 49.805) ccw
  arc A427 (-63.2315, 49.5618) -> (-63.1389, 49.8696) centre (-64.1304, 50) ccw
  arc A428 (-62.9902, 50) -> (-63.1389, 49.8696) centre (-62.9902, 49.85) ccw
  line L73 (-62.9902, 50) -> (-62.4709, 50)
  arc A429 (-62.3222, 49.8696) -> (-62.4709, 50) centre (-62.4709, 49.85) ccw
  arc A430 (-62.3222, 49.8696) -> (-62.2296, 49.5618) centre (-61.3307, 50) ccw
  arc A431 (-62.2296, 49.5618) -> (-61.7306, 49.25) centre (-61.7307, 49.805) ccw
  arc A432 (-61.7306, 49.25) -> (-61.2315, 49.5618) centre (-61.7304, 49.805) ccw
  arc A433 (-61.2315, 49.5618) -> (-61.1389, 49.8696) centre (-62.1304, 50) ccw
  arc A434 (-60.9902, 50) -> (-61.1389, 49.8696) centre (-60.9902, 49.85) ccw
  line L74 (-60.9902, 50) -> (-60.4709, 50)
  arc A435 (-60.3222, 49.8696) -> (-60.4709, 50) centre (-60.4709, 49.85) ccw
  arc A436 (-60.3222, 49.8696) -> (-60.2296, 49.5618) centre (-59.3307, 50) ccw
  arc A437 (-60.2296, 49.5618) -> (-59.7306, 49.25) centre (-59.7307, 49.805) ccw
  arc A438 (-59.7306, 49.25) -> (-59.2315, 49.5618) centre (-59.7304, 49.805) ccw
  arc A439 (-59.2315, 49.5618) -> (-59.1389, 49.8696) centre (-60.1304, 50) ccw
  arc A440 (-58.9902, 50) -> (-59.1389, 49.8696) centre (-58.9902, 49.85) ccw
  line L75 (-58.9902, 50) -> (-58.4709, 50)
  arc A441 (-58.3222, 49.8696) -> (-58.4709, 50) centre (-58.4709, 49.85) ccw
  arc A442 (-58.3222, 49.8696) -> (-58.2296, 49.5618) centre (-57.3307, 50) ccw
  arc A443 (-58.2296, 49.5618) -> (-57.7306, 49.25) centre (-57.7307, 49.805) ccw
  arc A444 (-57.7306, 49.25) -> (-57.2315, 49.5618) centre (-57.7304, 49.805) ccw
  arc A445 (-57.2315, 49.5618) -> (-57.1389, 49.8696) centre (-58.1304, 50) ccw
  arc A446 (-56.9902, 50) -> (-57.1389, 49.8696) centre (-56.9902, 49.85) ccw
  line L76 (-56.9902, 50) -> (-56.4709, 50)
  arc A447 (-56.3222, 49.8696) -> (-56.4709, 50) centre (-56.4709, 49.85) ccw
  arc A448 (-56.3222, 49.8696) -> (-56.2296, 49.5618) centre (-55.3307, 50) ccw
  arc A449 (-56.2296, 49.5618) -> (-55.7306, 49.25) centre (-55.7307, 49.805) ccw
  arc A450 (-55.7306, 49.25) -> (-55.2315, 49.5618) centre (-55.7304, 49.805) ccw
  arc A451 (-55.2315, 49.5618) -> (-55.1389, 49.8696) centre (-56.1304, 50) ccw
  arc A452 (-54.9902, 50) -> (-55.1389, 49.8696) centre (-54.9902, 49.85) ccw
  line L77 (-54.9902, 50) -> (-54.4709, 50)
  arc A453 (-54.3222, 49.8696) -> (-54.4709, 50) centre (-54.4709, 49.85) ccw
  arc A454 (-54.3222, 49.8696) -> (-54.2296, 49.5618) centre (-53.3307, 50) ccw
  arc A455 (-54.2296, 49.5618) -> (-53.7306, 49.25) centre (-53.7307, 49.805) ccw
  arc A456 (-53.7306, 49.25) -> (-53.2315, 49.5618) centre (-53.7304, 49.805) ccw
  arc A457 (-53.2315, 49.5618) -> (-53.1389, 49.8696) centre (-54.1304, 50) ccw
  arc A458 (-52.9902, 50) -> (-53.1389, 49.8696) centre (-52.9902, 49.85) ccw
  line L78 (-52.9902, 50) -> (-52.4709, 50)
  arc A459 (-52.3222, 49.8696) -> (-52.4709, 50) centre (-52.4709, 49.85) ccw
  arc A460 (-52.3222, 49.8696) -> (-52.2296, 49.5618) centre (-51.3307, 50) ccw
  arc A461 (-52.2296, 49.5618) -> (-51.7306, 49.25) centre (-51.7307, 49.805) ccw
  arc A462 (-51.7306, 49.25) -> (-51.2315, 49.5618) centre (-51.7304, 49.805) ccw
  arc A463 (-51.2315, 49.5618) -> (-51.1389, 49.8696) centre (-52.1304, 50) ccw
  arc A464 (-50.9902, 50) -> (-51.1389, 49.8696) centre (-50.9902, 49.85) ccw
  line L79 (-50.9902, 50) -> (-50.4709, 50)
  arc A465 (-50.3222, 49.8696) -> (-50.4709, 50) centre (-50.4709, 49.85) ccw
  arc A466 (-50.3222, 49.8696) -> (-50.2296, 49.5618) centre (-49.3307, 50) ccw
  arc A467 (-50.2296, 49.5618) -> (-49.7306, 49.25) centre (-49.7307, 49.805) ccw
  arc A468 (-49.7306, 49.25) -> (-49.2315, 49.5618) centre (-49.7304, 49.805) ccw
  arc A469 (-49.2315, 49.5618) -> (-49.1389, 49.8696) centre (-50.1304, 50) ccw
  arc A470 (-48.9902, 50) -> (-49.1389, 49.8696) centre (-48.9902, 49.85) ccw
  line L80 (-48.9902, 50) -> (-48.4709, 50)
  arc A471 (-48.3222, 49.8696) -> (-48.4709, 50) centre (-48.4709, 49.85) ccw
  arc A472 (-48.3222, 49.8696) -> (-48.2296, 49.5618) centre (-47.3307, 50) ccw
  arc A473 (-48.2296, 49.5618) -> (-47.7306, 49.25) centre (-47.7307, 49.805) ccw
  arc A474 (-47.7306, 49.25) -> (-47.2315, 49.5618) centre (-47.7304, 49.805) ccw
  arc A475 (-47.2315, 49.5618) -> (-47.1389, 49.8696) centre (-48.1304, 50) ccw
  arc A476 (-46.9902, 50) -> (-47.1389, 49.8696) centre (-46.9902, 49.85) ccw
  line L81 (-46.9902, 50) -> (-46.4709, 50)
  arc A477 (-46.3222, 49.8696) -> (-46.4709, 50) centre (-46.4709, 49.85) ccw
  arc A478 (-46.3222, 49.8696) -> (-46.2296, 49.5618) centre (-45.3307, 50) ccw
  arc A479 (-46.2296, 49.5618) -> (-45.7306, 49.25) centre (-45.7307, 49.805) ccw
  arc A480 (-45.7306, 49.25) -> (-45.2315, 49.5618) centre (-45.7304, 49.805) ccw
  arc A481 (-45.2315, 49.5618) -> (-45.1389, 49.8696) centre (-46.1304, 50) ccw
  arc A482 (-44.9902, 50) -> (-45.1389, 49.8696) centre (-44.9902, 49.85) ccw
  line L82 (-44.9902, 50) -> (-44.4709, 50)
  arc A483 (-44.3222, 49.8696) -> (-44.4709, 50) centre (-44.4709, 49.85) ccw
  arc A484 (-44.3222, 49.8696) -> (-44.2296, 49.5618) centre (-43.3307, 50) ccw
  arc A485 (-44.2296, 49.5618) -> (-43.7306, 49.25) centre (-43.7307, 49.805) ccw
  arc A486 (-43.7306, 49.25) -> (-43.2315, 49.5618) centre (-43.7304, 49.805) ccw
  arc A487 (-43.2315, 49.5618) -> (-43.1389, 49.8696) centre (-44.1304, 50) ccw
  arc A488 (-42.9902, 50) -> (-43.1389, 49.8696) centre (-42.9902, 49.85) ccw
  line L83 (-42.9902, 50) -> (-42.4709, 50)
  arc A489 (-42.3222, 49.8696) -> (-42.4709, 50) centre (-42.4709, 49.85) ccw
  arc A490 (-42.3222, 49.8696) -> (-42.2296, 49.5618) centre (-41.3307, 50) ccw
  arc A491 (-42.2296, 49.5618) -> (-41.7306, 49.25) centre (-41.7307, 49.805) ccw
  arc A492 (-41.7306, 49.25) -> (-41.2315, 49.5618) centre (-41.7304, 49.805) ccw
  arc A493 (-41.2315, 49.5618) -> (-41.1389, 49.8696) centre (-42.1304, 50) ccw
  arc A494 (-40.9902, 50) -> (-41.1389, 49.8696) centre (-40.9902, 49.85) ccw
  line L84 (-40.9902, 50) -> (-40.4709, 50)
  arc A495 (-40.3222, 49.8696) -> (-40.4709, 50) centre (-40.4709, 49.85) ccw
  arc A496 (-40.3222, 49.8696) -> (-40.2296, 49.5618) centre (-39.3307, 50) ccw
  arc A497 (-40.2296, 49.5618) -> (-39.7306, 49.25) centre (-39.7307, 49.805) ccw
  arc A498 (-39.7306, 49.25) -> (-39.2315, 49.5618) centre (-39.7304, 49.805) ccw
  arc A499 (-39.2315, 49.5618) -> (-39.1389, 49.8696) centre (-40.1304, 50) ccw
  arc A500 (-38.9902, 50) -> (-39.1389, 49.8696) centre (-38.9902, 49.85) ccw
  line L85 (-38.9902, 50) -> (-38.4709, 50)
  arc A501 (-38.3222, 49.8696) -> (-38.4709, 50) centre (-38.4709, 49.85) ccw
  arc A502 (-38.3222, 49.8696) -> (-38.2296, 49.5618) centre (-37.3307, 50) ccw
  arc A503 (-38.2296, 49.5618) -> (-37.7306, 49.25) centre (-37.7307, 49.805) ccw
  arc A504 (-37.7306, 49.25) -> (-37.2315, 49.5618) centre (-37.7304, 49.805) ccw
  arc A505 (-37.2315, 49.5618) -> (-37.1389, 49.8696) centre (-38.1304, 50) ccw
  arc A506 (-36.9902, 50) -> (-37.1389, 49.8696) centre (-36.9902, 49.85) ccw
  line L86 (-36.9902, 50) -> (-36.4709, 50)
  arc A507 (-36.3222, 49.8696) -> (-36.4709, 50) centre (-36.4709, 49.85) ccw
  arc A508 (-36.3222, 49.8696) -> (-36.2296, 49.5618) centre (-35.3307, 50) ccw
  arc A509 (-36.2296, 49.5618) -> (-35.7306, 49.25) centre (-35.7307, 49.805) ccw
  arc A510 (-35.7306, 49.25) -> (-35.2315, 49.5618) centre (-35.7304, 49.805) ccw
  arc A511 (-35.2315, 49.5618) -> (-35.1389, 49.8696) centre (-36.1304, 50) ccw
  arc A512 (-34.9902, 50) -> (-35.1389, 49.8696) centre (-34.9902, 49.85) ccw
  line L87 (-34.9902, 50) -> (-34.4709, 50)
  arc A513 (-34.3222, 49.8696) -> (-34.4709, 50) centre (-34.4709, 49.85) ccw
  arc A514 (-34.3222, 49.8696) -> (-34.2296, 49.5618) centre (-33.3307, 50) ccw
  arc A515 (-34.2296, 49.5618) -> (-33.7306, 49.25) centre (-33.7307, 49.805) ccw
  arc A516 (-33.7306, 49.25) -> (-33.2315, 49.5618) centre (-33.7304, 49.805) ccw
  arc A517 (-33.2315, 49.5618) -> (-33.1389, 49.8696) centre (-34.1304, 50) ccw
  arc A518 (-32.9902, 50) -> (-33.1389, 49.8696) centre (-32.9902, 49.85) ccw
  line L88 (-32.9902, 50) -> (-32.4709, 50)
  arc A519 (-32.3222, 49.8696) -> (-32.4709, 50) centre (-32.4709, 49.85) ccw
  arc A520 (-32.3222, 49.8696) -> (-32.2296, 49.5618) centre (-31.3307, 50) ccw
  arc A521 (-32.2296, 49.5618) -> (-31.7306, 49.25) centre (-31.7307, 49.805) ccw
  arc A522 (-31.7306, 49.25) -> (-31.2315, 49.5618) centre (-31.7304, 49.805) ccw
  arc A523 (-31.2315, 49.5618) -> (-31.1389, 49.8696) centre (-32.1304, 50) ccw
  arc A524 (-30.9902, 50) -> (-31.1389, 49.8696) centre (-30.9902, 49.85) ccw
  line L89 (-30.9902, 50) -> (-30.4709, 50)
  arc A525 (-30.3222, 49.8696) -> (-30.4709, 50) centre (-30.4709, 49.85) ccw
  arc A526 (-30.3222, 49.8696) -> (-30.2296, 49.5618) centre (-29.3307, 50) ccw
  arc A527 (-30.2296, 49.5618) -> (-29.7306, 49.25) centre (-29.7307, 49.805) ccw
  arc A528 (-29.7306, 49.25) -> (-29.2315, 49.5618) centre (-29.7304, 49.805) ccw
  arc A529 (-29.2315, 49.5618) -> (-29.1389, 49.8696) centre (-30.1304, 50) ccw
  arc A530 (-28.9902, 50) -> (-29.1389, 49.8696) centre (-28.9902, 49.85) ccw
  line L90 (-28.9902, 50) -> (-28.4709, 50)
  arc A531 (-28.3222, 49.8696) -> (-28.4709, 50) centre (-28.4709, 49.85) ccw
  arc A532 (-28.3222, 49.8696) -> (-28.2296, 49.5618) centre (-27.3307, 50) ccw
  arc A533 (-28.2296, 49.5618) -> (-27.7306, 49.25) centre (-27.7307, 49.805) ccw
  arc A534 (-27.7306, 49.25) -> (-27.2315, 49.5618) centre (-27.7304, 49.805) ccw
  arc A535 (-27.2315, 49.5618) -> (-27.1389, 49.8696) centre (-28.1304, 50) ccw
  arc A536 (-26.9902, 50) -> (-27.1389, 49.8696) centre (-26.9902, 49.85) ccw
  line L91 (-26.9902, 50) -> (-26.4709, 50)
  arc A537 (-26.3222, 49.8696) -> (-26.4709, 50) centre (-26.4709, 49.85) ccw
  arc A538 (-26.3222, 49.8696) -> (-26.2296, 49.5618) centre (-25.3307, 50) ccw
  arc A539 (-26.2296, 49.5618) -> (-25.7306, 49.25) centre (-25.7307, 49.805) ccw
  arc A540 (-25.7306, 49.25) -> (-25.2315, 49.5618) centre (-25.7304, 49.805) ccw
  arc A541 (-25.2315, 49.5618) -> (-25.1389, 49.8696) centre (-26.1304, 50) ccw
  arc A542 (-24.9902, 50) -> (-25.1389, 49.8696) centre (-24.9902, 49.85) ccw
  line L92 (-24.9902, 50) -> (-24.4709, 50)
  arc A543 (-24.3222, 49.8696) -> (-24.4709, 50) centre (-24.4709, 49.85) ccw
  arc A544 (-24.3222, 49.8696) -> (-24.2296, 49.5618) centre (-23.3307, 50) ccw
  arc A545 (-24.2296, 49.5618) -> (-23.7306, 49.25) centre (-23.7307, 49.805) ccw
  arc A546 (-23.7306, 49.25) -> (-23.2315, 49.5618) centre (-23.7304, 49.805) ccw
  arc A547 (-23.2315, 49.5618) -> (-23.1389, 49.8696) centre (-24.1304, 50) ccw
  arc A548 (-22.9902, 50) -> (-23.1389, 49.8696) centre (-22.9902, 49.85) ccw
  line L93 (-22.9902, 50) -> (-22.4709, 50)
  arc A549 (-22.3222, 49.8696) -> (-22.4709, 50) centre (-22.4709, 49.85) ccw
  arc A550 (-22.3222, 49.8696) -> (-22.2296, 49.5618) centre (-21.3307, 50) ccw
  arc A551 (-22.2296, 49.5618) -> (-21.7306, 49.25) centre (-21.7307, 49.805) ccw